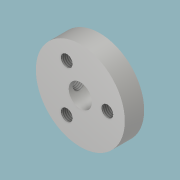
# Autodesk Inventor part: 6mm Mounting Hub, thin
Saved by Autodesk Inventor 2017 SP1 (Build 210196100, 196)
## iProperties
Created: 2016-03-07
Part Number: 6mm Mounting Hub, thin
Material: Aluminum 6061
Description: STEP AP214
Document SubType Name: Modeling
Designer: Zach
Density: 2.7 g/cm^3
Appearance: Aluminum - Flat
Sending System: SolidWorks 2015
Preprocessor: SwSTEP 2.0
Title: hub02-6mm.step
Revision Number: ANY
Autodesk Inventor part; units mm, degrees
ref_plane "YZ Plane" through (0, 0, 0) normal (1, 0, 0) x (0, 1, 0)
ref_plane "XZ Plane" through (0, 0, 0) normal (0, 1, 0) x (-1, 0, 0)
ref_plane "XY Plane" through (0, 0, 0) normal (0, 0, 1) x (1, 0, 0)
sketch "Sketch3" plane through (0, 0, 0) normal (0, 0, 1) x (1, 0, 0)
  circle A0 centre (0, 0) radius 11.5
  circle A1 centre (0, 0) radius 3
  circle A2 centre (7, 0) radius 1.5
  circle A3 centre (3.5, 6.0622) radius 1.5
  circle A4 centre (-3.5, 6.0622) radius 1.5
  circle A5 centre (-7, 0) radius 1.5
  circle A6 centre (-3.5, -6.0622) radius 1.5
  circle A7 centre (3.5, -6.0622) radius 1.5
  dimension "d0" = 23
  dimension "d1" = 6
  dimension "d4" = 3
  dimension "d5" = 7
  dimension "d12" = 360
  constraints: 8 centre point, 2 coincident, 1 horizontal alignment, 13 other
  measures "d0" diameter of A0
  measures "d1" diameter of A1
  measures "d4" diameter of A2
  measures "d5" distance of point (0, 0) A2.centre
extrude "Extrusion1" add sketch "Sketch3" along normal blind 5 contours A0 | A3 | A5 | A7
sketch "Sketch4" plane through (0, 0, 0) normal (1, 0, 0) x (0, 1, 0)
  line L0 (-11.5, 0) -> (11.5, 0) projected
  line L1 (-3, 5) -> (3, 5) projected
  line L2 (3, 0) -> (-3, 0) projected
  circle A0 centre (0, 2.5) radius 1.5
  line L3 (3, 0) -> (3, 5) projected
  point P0 (0, 0)
  point P1 (0, 0)
  point P2 (3, 2.5)
  dimension "d14" = 3
  constraints: 2 midpoint, 1 centre point, 1 horizontal alignment, 1 vertical alignment
  measures "d14" diameter of A0
extrude "Extrusion2" cut sketch "Sketch4" against normal through all
thread "Thread1" size "M3x0.5" class "6H" standard "ANSI Metric M Profile" full length
thread "Thread2" size "M3x0.5" class "6H" standard "ANSI Metric M Profile" full length
thread "Thread3" size "M3x0.5" class "6H" standard "ANSI Metric M Profile" full length
thread "Thread4" size "M3x0.5" class "6H" standard "ANSI Metric M Profile" full length
equation "\"d15\" = d14"
body "Solid2"
